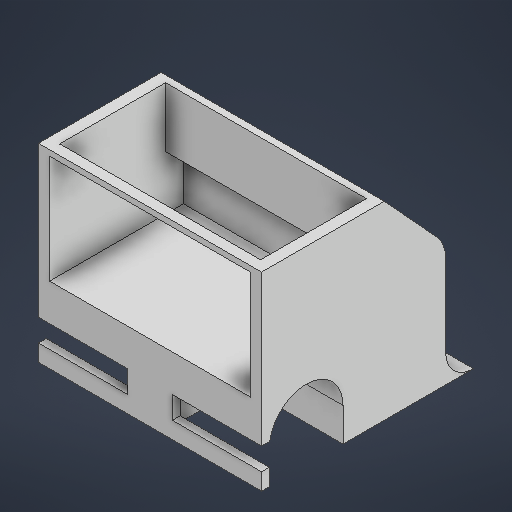
# Autodesk Inventor part: mini sumô rascunho v2
Saved by Autodesk Inventor 2026.1 (Build 301233000, 233)
## iProperties
Created: 2025-11-07
Part Number: mini sumô rascunho v2
Material: Genérico
Document SubType Name: Modeling
Designer: panto
Density: 1 g/cm^3
Appearance: Padrão
Author: panto
Autodesk Inventor part; units mm, degrees
ref_plane "YZ Plane" through (0, 0, 0) normal (1, 0, 0) x (0, 1, 0)
ref_plane "XZ Plane" through (0, 0, 0) normal (0, 1, 0) x (-1, 0, 0)
ref_plane "XY Plane" through (0, 0, 0) normal (0, 0, 1) x (1, 0, 0)
sketch "Esboço1" plane through (0, 0, 0) normal (0, 1, 0) x (-1, 0, 0)
  line L0 (0, 0) -> (100, 0)
  line L1 (100, 0) -> (100, -100)
  line L2 (100, -100) -> (0, -100)
  line L3 (0, -100) -> (0, 0)
  dimension "d0" = 100
  dimension "d1" = 100
  constraints: 8 end point, 2 parallel, 1 horizontal, 1 perpendicular
  measures "d0" distance of L1.end L2.end
  measures "d1" distance of L0.end L1.end
extrude "Extrusão1" add sketch "Esboço1" along normal blind 85
sketch "Esboço2" plane through (0, 0, 0) normal (1, 0, 0) x (0, 0, -1)
  line L0 (100, 0) -> (0, 0) projected
  line L1 (0, 0) -> (20, 0)
  circle A0 centre (20, 15) radius 15
  line L2 (35, 15) -> (35, 0)
  line L3 (5, 15) -> (5, 0)
  line L4 (100, 85) -> (0, 85) projected
  line L5 (100, 0) -> (100, 85) projected
  line L6 (0, 85) -> (25, 85)
  line L7 (100, 10) -> (100, 0)
  line L8 (100, 0) -> (95, 0)
  line L9 (0, 0) -> (0, 85)
  line L10 (100, 0) -> (89.5, 0)
  line L11 (82.5, 12.5) -> (82.5, 49.1652)
  line L12 (0, 85) -> (55, 85)
  line L13 (100, 85) -> (100, 0)
  line L14 (100, 0) -> (0, 0)
  line L15 (0, 0) -> (0, 85)
  line L16 (78.5573, 59.3011) -> (55, 85)
  arc A1 (82.5, 49.1652) -> (78.5573, 59.3011) centre (67.5, 49.1652) ccw
  arc A2 (82.5, 12.5) -> (95, 0) centre (95, 12.5) ccw
  point P0 (82.5, 0)
  point P1 (82.5, 85)
  point P2 (5, 0)
  dimension "d6" = 30
  dimension "d8" = 17.5
  dimension "d11" = 15
  dimension "d12" = 12.5
  constraints: 28 end point, 10 point on line, 6 point on circle, 5 tangent, 4 parallel, 4 perpendicular, 3 centre point, 2 horizontal, 1 vertical
  measures "d6" diameter of A0
  measures "d8" distance of L0.start point (82.5, 0)
  measures "d11" radius of A1
  measures "d12" radius of A2
extrude "Extrusão2" cut sketch "Esboço2" against normal blind 100 contours L0 A2 L11 A1 L16 L4 L5
extrude "Extrusão3" cut sketch "Esboço2" against normal blind 45 contours L0 A0 L2 | L0 L3 A0 | A0
sketch "Esboço3" plane through (-100, 0, 0) normal (-1, 0, 0) x (0, 0, 1)
  arc A0 (-5, 15) -> (-35, 15) centre (-20, 15) ccw projected
  line L0 (-20, 15) -> (-20, 0)
  line L1 (-95, 0) -> (0, 0) projected
  circle A1 centre (-20, 15) radius 15
  line L2 (-35, 15) -> (-35, -0.9881)
  line L3 (-5, 0) -> (-5, 15) projected
  line L4 (-5, 15) -> (-5, 0)
  line L5 (-35, 0) -> (-5, 0)
  constraints: 8 end point, 3 point on line, 2 collinear, 2 tangent, 1 centre point, 1 coincident, 1 perpendicular, 1 vertical
extrude "Extrusão4" cut sketch "Esboço3" against normal blind 45
sketch "Esboço4" plane through (-100, 0, 0) normal (0, 0, 1) x (1, 0, 0)
  line L0 (0, 0) -> (0, 12.5) projected
  line L1 (0, 12.5) -> (0, 17.5)
  line L2 (0, 49.1652) -> (0, 12.5) projected
  line L3 (0, 17.5) -> (0, 7.5)
  line L4 (0, 17.5) -> (40, 17.5)
  line L5 (45, 15) -> (45, 30) projected
  line L6 (40, 17.5) -> (40, 7.5)
  line L7 (40, 7.5) -> (0, 7.5)
  line L8 (100, 12.5) -> (100, 49.1652) projected
  line L9 (100, 17.5) -> (100, 7.5)
  line L10 (100, 7.5) -> (60, 7.5)
  line L11 (60, 7.5) -> (60, 17.5)
  line L12 (60, 17.5) -> (100, 17.5)
  line L13 (45, 30) -> (45, 34)
  line L14 (45, 34) -> (95, 34)
  line L15 (45, 34) -> (5, 34)
  line L16 (5, 34) -> (95, 34)
  line L17 (5, 34) -> (5, 82.5)
  line L18 (5, 82.5) -> (95, 82.5)
  line L19 (95, 82.5) -> (95, 34)
  line L20 (5, 34) -> (5, 61.5)
  line L21 (5, 34) -> (5, 58.25)
  line L22 (5, 58.25) -> (95, 58.25)
  line L23 (95, 58.25) -> (95, 34)
  line L24 (95, 34) -> (5, 34)
  point P0 (100, 0)
  dimension "d20" = 10
  dimension "d22" = 40
  dimension "d27" = 48.5
  constraints: 42 end point, 9 perpendicular, 5 point on line, 4 collinear, 1 horizontal, 1 midpoint, 1 parallel, 1 vertical
  measures "d20" distance of L1.end L3.end
  measures "d22" distance of L9.end L10.end
  measures "d27" distance of L15.end L17.end
extrude "Extrusão5" cut sketch "Esboço4" against normal blind 10 contours L0 L1 L4 L6 L7 | L9 L10 L11 L12 L8
extrude "Extrusão6" cut sketch "Esboço4" against normal blind 52 contours L22 L17 L18 L19
extrude "Extrusão7" cut sketch "Esboço4" against normal blind 60 contours L15 L17 L22 L19 L14
sketch "Esboço5" plane through (0, 85, 0) normal (0, 1, 0) x (1, 0, 0)
  line L0 (-95, 0) -> (-95, 52) projected
  line L1 (-95, 4.5451) -> (-95, 52)
  line L2 (-5, 0) -> (-5, 52) projected
  line L3 (-95, 52) -> (-5, 52)
  line L4 (-5, 52) -> (-5, 4.5451)
  line L5 (-5, 4.5451) -> (-95, 4.5451)
  point P0 (0, 0)
  constraints: 8 end point, 3 perpendicular, 1 collinear, 1 point on line
extrude "Extrusão8" cut sketch "Esboço5" against normal blind 10.75
sketch "Esboço6" plane through (-100, 12.5, -82.5) normal (-1, 0, 0) x (0, 0, 1)
  arc A0 (77.2902, 5) -> (47.5, 2.5) centre (62.5, 2.5) ccw projected
  circle A1 centre (62.5, 2.5) radius 16.5
  line L0 (46, 2.5) -> (46, -12.5)
  line L1 (79, 2.5) -> (79, -12.5)
  line L2 (82.5, 5) -> (82.5, -5) projected
  line L3 (46, -12.5) -> (79, -12.5)
  line L4 (77.5, -12.5) -> (82.5, -12.5) projected
  dimension "d37" = 33
  constraints: 6 end point, 2 point on circle, 2 tangent, 1 centre point, 1 coincident, 1 collinear, 1 parallel, 1 vertical
  measures "d37" diameter of A1
extrude "Extrusão9" cut sketch "Esboço6" against normal blind 45 contours A1 L3 | L1 L3 A1 | A1 L3 L0 picked at (60.7652, -1.3921)
sketch "Esboço7" plane through (0, 12.5, -82.5) normal (1, 0, 0) x (0, 0, -1)
  arc A0 (-46, 2.5) -> (-79, 2.5) centre (-62.5, 2.5) ccw projected
  circle A1 centre (-62.5, 2.5) radius 16.5
  line L0 (-79, -12.5) -> (-82.5, -12.5) projected
  line L1 (-79, 2.5) -> (-79, -12.5)
  line L2 (-79, -12.5) -> (-46, -12.5)
  line L3 (-46, -12.5) -> (-46, 2.5)
  dimension "d40" = 33
  constraints: 6 end point, 1 centre point, 1 coincident, 1 perpendicular, 1 tangent, 1 vertical
  measures "d40" diameter of A1
extrude "Extrusão10" cut sketch "Esboço7" against normal blind 45 contours A1 L2 A0 | L3 L2 A1 | A1 L2 L1
